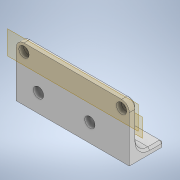
# Autodesk Inventor part: bracket_t265nd455_external
Saved by Autodesk Inventor 2022.1 (Build 261234000, 234)
## iProperties
Created: 2021-08-20
Part Number: bracket_t265nd455_external
Material: Generic
Document SubType Name: Modeling
Designer: 오유진
Density: 1 g/cm^3
Appearance: Default
Author: 오유진
Autodesk Inventor part; units mm, degrees
(part 1 of 2)
ref_plane "YZ Plane" through (0, 0, 0) normal (1, 0, 0) x (0, 1, 0)
ref_plane "XZ Plane" through (0, 0, 0) normal (0, 1, 0) x (-1, 0, 0)
ref_plane "XY Plane" through (0, 0, 0) normal (0, 0, 1) x (1, 0, 0)
ref_plane "Work Plane3" through (-46, 39.5, 21) normal (0, 0, 1) x (1, 0, 0)
sketch "Sketch5" plane through (-46, 39.5, 21) normal (0, 0, 1) x (1, 0, 0)
  line L0 (41.5, 10.3889) -> (-41.5, 10.3889) projected
  spline S0 degree 3 poles (-52.6944, 8.9971) (-52.5847, 9.0604) (-52.4738, 9.1218) (-52.3618, 9.181) (-52.263, 9.2333) (-52.1634, 9.2839) (-52.063, 9.3329) (-51.9718, 9.3773) (-51.8801, 9.4203) (-51.7876, 9.4618) (-51.6999, 9.5013) (-51.6116, 9.5395) (-51.5228, 9.5763) (-51.435, 9.6128) (-51.3468, 9.6479) (-51.258, 9.6817) (-51.1696, 9.7154) (-51.0807, 9.7479) (-50.9913, 9.779) (-50.9017, 9.8102) (-50.8117, 9.8401) (-50.7213, 9.8687) (-50.6307, 9.8973) (-50.5398, 9.9246) (-50.4485, 9.9506) (-50.3572, 9.9766) (-50.2655, 10.0013) (-50.1736, 10.0246) (-50.0816, 10.0479) (-49.9892, 10.0699) (-49.8966, 10.0905) (-49.8038, 10.1112) (-49.7107, 10.1306) (-49.6173, 10.1486) (-49.5236, 10.1666) (-49.4296, 10.1834) (-49.3352, 10.1989) (-49.2404, 10.2144) (-49.1453, 10.2287) (-49.0498, 10.2418) (-48.9539, 10.255) (-48.8576, 10.267) (-48.7611, 10.2779) (-48.6642, 10.2888) (-48.567, 10.2987) (-48.4696, 10.3076) (-48.3718, 10.3166) (-48.2737, 10.3245) (-48.1754, 10.3316) (-48.0763, 10.3388) (-47.977, 10.345) (-47.8775, 10.3505) (-47.7769, 10.3561) (-47.6762, 10.3609) (-47.5754, 10.365) (-47.4739, 10.3691) (-47.3722, 10.3726) (-47.2704, 10.3755) (-47.1677, 10.3785) (-47.065, 10.3808) (-46.9621, 10.3827) (-46.8576, 10.3847) (-46.753, 10.3862) (-46.6483, 10.3873) (-46.5422, 10.3884) (-46.436, 10.3892) (-46.3298, 10.3897) (-46.2236, 10.3902) (-46.1173, 10.3905) (-46.011, 10.3906) (-45.9052, 10.3907) (-45.7994, 10.3907) (-45.6934, 10.3906) (-45.5876, 10.3905) (-45.4817, 10.3903) (-45.3757, 10.3902) (-45.2696, 10.39) (-45.1635, 10.3899) (-45.0574, 10.3898) (-44.9513, 10.3897) (-44.8452, 10.3896) (-44.7391, 10.3896) (-44.6331, 10.3895) (-44.5271, 10.3895) (-44.4211, 10.3895) (-44.3151, 10.3894) (-44.209, 10.3894) (-44.103, 10.3894) (-43.9969, 10.3893) (-43.8907, 10.3893) (-43.7846, 10.3893) (-43.6785, 10.3892) (-43.5724, 10.3892) (-43.4663, 10.3891) (-43.3604, 10.3891) (-43.2545, 10.3891) (-43.1486, 10.389) (-43.0427, 10.389) (-42.9368, 10.389) (-42.831, 10.389) (-42.7244, 10.3889) (-42.6178, 10.3889) (-42.5112, 10.3889) (-42.4028, 10.3889) (-42.2944, 10.3889) (-42.186, 10.3889) (-42.0747, 10.3889) (-41.9634, 10.3889) (-41.8521, 10.3889) (-41.7347, 10.3889) (-41.6174, 10.3889) (-41.5, 10.3889) knots 0 0 0 0 0.033772 0.033772 0.033772 0.063568 0.063568 0.063568 0.090608 0.090608 0.090608 0.116279 0.116279 0.116279 0.141638 0.141638 0.141638 0.166894 0.166894 0.166894 0.192211 0.192211 0.192211 0.217549 0.217549 0.217549 0.242877 0.242877 0.242877 0.268207 0.268207 0.268207 0.293578 0.293578 0.293578 0.319038 0.319038 0.319038 0.344627 0.344627 0.344627 0.370358 0.370358 0.370358 0.3962 0.3962 0.3962 0.422164 0.422164 0.422164 0.448361 0.448361 0.448361 0.47483 0.47483 0.47483 0.501477 0.501477 0.501477 0.528339 0.528339 0.528339 0.555617 0.555617 0.555617 0.583244 0.583244 0.583244 0.610845 0.610845 0.610845 0.638286 0.638286 0.638286 0.665706 0.665706 0.665706 0.693157 0.693157 0.693157 0.720597 0.720597 0.720597 0.748024 0.748024 0.748024 0.775467 0.775467 0.775467 0.802931 0.802931 0.802931 0.830389 0.830389 0.830389 0.857797 0.857797 0.857797 0.885191 0.885191 0.885191 0.912774 0.912774 0.912774 0.940826 0.940826 0.940826 0.969629 0.969629 0.969629 1 1 1 1 projected
  arc A0 (-52.6944, 8.9971) -> (-52.6944, -8.9971) centre (-47.5, 0) ccw projected
  spline S1 degree 3 poles (-41.5, -10.3889) (-41.6309, -10.3889) (-41.7619, -10.3889) (-41.8928, -10.3889) (-42.0134, -10.3889) (-42.134, -10.3889) (-42.2546, -10.3889) (-42.3674, -10.3889) (-42.4802, -10.3889) (-42.593, -10.3889) (-42.7013, -10.3889) (-42.8095, -10.3889) (-42.9178, -10.389) (-43.0247, -10.389) (-43.1315, -10.389) (-43.2384, -10.3891) (-43.3448, -10.3891) (-43.4512, -10.3891) (-43.5575, -10.3892) (-43.6641, -10.3892) (-43.7706, -10.3893) (-43.8771, -10.3893) (-43.9838, -10.3893) (-44.0904, -10.3894) (-44.197, -10.3894) (-44.3036, -10.3894) (-44.4102, -10.3895) (-44.5167, -10.3895) (-44.6232, -10.3895) (-44.7297, -10.3896) (-44.8363, -10.3896) (-44.9428, -10.3897) (-45.0493, -10.3898) (-45.1557, -10.3899) (-45.2623, -10.39) (-45.3688, -10.3902) (-45.4753, -10.3903) (-45.582, -10.3905) (-45.6885, -10.3906) (-45.795, -10.3906) (-45.9015, -10.3907) (-46.008, -10.3906) (-46.1144, -10.3904) (-46.2206, -10.3902) (-46.3267, -10.3898) (-46.4327, -10.3891) (-46.5381, -10.3884) (-46.6434, -10.3875) (-46.7486, -10.3861) (-46.8525, -10.3847) (-46.9563, -10.383) (-47.06, -10.3808) (-47.1622, -10.3786) (-47.2642, -10.3759) (-47.366, -10.3726) (-47.4669, -10.3694) (-47.5677, -10.3656) (-47.6683, -10.361) (-47.7686, -10.3565) (-47.8687, -10.3513) (-47.9687, -10.3453) (-48.068, -10.3393) (-48.1671, -10.3325) (-48.266, -10.3248) (-48.3638, -10.3172) (-48.4615, -10.3087) (-48.5589, -10.2992) (-48.6558, -10.2897) (-48.7525, -10.2792) (-48.8489, -10.2677) (-48.9453, -10.2561) (-49.0414, -10.2434) (-49.1372, -10.2295) (-49.2326, -10.2156) (-49.3277, -10.2005) (-49.4226, -10.1842) (-49.5168, -10.1679) (-49.6108, -10.1503) (-49.7044, -10.1314) (-49.7979, -10.1125) (-49.891, -10.0923) (-49.9839, -10.0707) (-50.0768, -10.0491) (-50.1695, -10.0261) (-50.2617, -10.0018) (-50.354, -9.9775) (-50.4459, -9.9518) (-50.5374, -9.9249) (-50.6288, -9.8979) (-50.7199, -9.8696) (-50.8106, -9.84) (-50.9012, -9.8104) (-50.9915, -9.7794) (-51.0812, -9.7472) (-51.1709, -9.715) (-51.2601, -9.6815) (-51.3487, -9.6466) (-51.4373, -9.6119) (-51.5253, -9.5758) (-51.6129, -9.5384) (-51.701, -9.5008) (-51.7885, -9.4619) (-51.8755, -9.4218) (-51.9643, -9.3808) (-52.0524, -9.3385) (-52.1399, -9.295) (-52.2303, -9.25) (-52.32, -9.2036) (-52.4091, -9.1559) (-52.505, -9.1045) (-52.6001, -9.0515) (-52.6944, -8.9971) knots 0 0 0 0 0.033887 0.033887 0.033887 0.06509 0.06509 0.06509 0.094285 0.094285 0.094285 0.122296 0.122296 0.122296 0.149952 0.149952 0.149952 0.177479 0.177479 0.177479 0.205048 0.205048 0.205048 0.232644 0.232644 0.232644 0.260224 0.260224 0.260224 0.287779 0.287779 0.287779 0.315326 0.315326 0.315326 0.34289 0.34289 0.34289 0.370486 0.370486 0.370486 0.398102 0.398102 0.398102 0.425677 0.425677 0.425677 0.453094 0.453094 0.453094 0.480189 0.480189 0.480189 0.506871 0.506871 0.506871 0.533301 0.533301 0.533301 0.559648 0.559648 0.559648 0.585815 0.585815 0.585815 0.611699 0.611699 0.611699 0.637449 0.637449 0.637449 0.663186 0.663186 0.663186 0.688825 0.688825 0.688825 0.714314 0.714314 0.714314 0.739759 0.739759 0.739759 0.765225 0.765225 0.765225 0.790684 0.790684 0.790684 0.816132 0.816132 0.816132 0.84159 0.84159 0.84159 0.867019 0.867019 0.867019 0.892415 0.892415 0.892415 0.917983 0.917983 0.917983 0.944058 0.944058 0.944058 0.970987 0.970987 0.970987 1 1 1 1 projected
  line L1 (-41.5, -10.3889) -> (41.5, -10.3889) projected
  spline S2 degree 3 poles (52.6945, -8.9971) (52.5838, -9.0609) (52.4721, -9.1228) (52.3592, -9.1824) (52.2597, -9.2351) (52.1593, -9.286) (52.0581, -9.3352) (51.9663, -9.3799) (51.8738, -9.4232) (51.7807, -9.465) (51.6923, -9.5047) (51.6033, -9.5431) (51.5138, -9.5801) (51.4253, -9.6167) (51.3363, -9.6521) (51.2468, -9.6861) (51.1577, -9.7199) (51.0681, -9.7525) (50.978, -9.7837) (50.8876, -9.8151) (50.7968, -9.8451) (50.7056, -9.8738) (50.6142, -9.9025) (50.5224, -9.93) (50.4302, -9.956) (50.3378, -9.9822) (50.2451, -10.0069) (50.152, -10.0304) (50.0588, -10.0538) (49.9652, -10.0759) (49.8713, -10.0966) (49.7771, -10.1174) (49.6826, -10.1368) (49.5878, -10.1549) (49.4925, -10.173) (49.3969, -10.1898) (49.3009, -10.2053) (49.2043, -10.2208) (49.1074, -10.2351) (49.0102, -10.2482) (48.9122, -10.2614) (48.8139, -10.2733) (48.7154, -10.2842) (48.6164, -10.2951) (48.5171, -10.3049) (48.4176, -10.3137) (48.3176, -10.3226) (48.2174, -10.3304) (48.117, -10.3374) (48.0156, -10.3445) (47.914, -10.3506) (47.8123, -10.356) (47.7094, -10.3614) (47.6064, -10.3661) (47.5032, -10.37) (47.3996, -10.374) (47.2959, -10.3773) (47.192, -10.3801) (47.0879, -10.3828) (46.9836, -10.385) (46.8791, -10.3867) (46.7737, -10.3885) (46.6682, -10.3898) (46.5625, -10.3907) (46.4561, -10.3916) (46.3496, -10.3922) (46.243, -10.3926) (46.1368, -10.3929) (46.0306, -10.393) (45.9243, -10.393) (45.8189, -10.3929) (45.7134, -10.3927) (45.6078, -10.3925) (45.5027, -10.3923) (45.3976, -10.392) (45.2924, -10.3917) (45.1874, -10.3914) (45.0824, -10.3912) (44.9774, -10.391) (44.8727, -10.3908) (44.7681, -10.3906) (44.6634, -10.3905) (44.5592, -10.3903) (44.4551, -10.3902) (44.3509, -10.3901) (44.2471, -10.39) (44.1434, -10.3899) (44.0396, -10.3898) (43.936, -10.3897) (43.8325, -10.3897) (43.7289, -10.3896) (43.6254, -10.3895) (43.5219, -10.3894) (43.4184, -10.3893) (43.315, -10.3893) (43.2117, -10.3892) (43.1083, -10.3891) (43.005, -10.3891) (42.9017, -10.389) (42.7984, -10.389) (42.6944, -10.389) (42.5904, -10.389) (42.4865, -10.3889) (42.3807, -10.3889) (42.275, -10.3889) (42.1693, -10.3889) (42.0607, -10.3889) (41.9521, -10.3889) (41.8435, -10.3889) (41.729, -10.3889) (41.6145, -10.3889) (41.5, -10.3889) knots 0 0 0 0 0.034033 0.034033 0.034033 0.064049 0.064049 0.064049 0.091284 0.091284 0.091284 0.117145 0.117145 0.117145 0.142696 0.142696 0.142696 0.168144 0.168144 0.168144 0.193662 0.193662 0.193662 0.219234 0.219234 0.219234 0.244842 0.244842 0.244842 0.270502 0.270502 0.270502 0.296244 0.296244 0.296244 0.322113 0.322113 0.322113 0.348164 0.348164 0.348164 0.37441 0.37441 0.37441 0.40079 0.40079 0.40079 0.427301 0.427301 0.427301 0.454074 0.454074 0.454074 0.481133 0.481133 0.481133 0.508306 0.508306 0.508306 0.53556 0.53556 0.53556 0.563073 0.563073 0.563073 0.590787 0.590787 0.590787 0.618371 0.618371 0.618371 0.645713 0.645713 0.645713 0.672935 0.672935 0.672935 0.700093 0.700093 0.700093 0.727156 0.727156 0.727156 0.754106 0.754106 0.754106 0.780956 0.780956 0.780956 0.807754 0.807754 0.807754 0.834538 0.834538 0.834538 0.861282 0.861282 0.861282 0.888009 0.888009 0.888009 0.914912 0.914912 0.914912 0.94227 0.94227 0.94227 0.970367 0.970367 0.970367 1 1 1 1 projected
  arc A1 (52.6944, -8.9971) -> (52.6944, 8.9971) centre (47.5, 0) ccw projected
  spline S3 degree 3 poles (41.5, 10.3889) (41.6279, 10.3889) (41.7557, 10.3889) (41.8836, 10.3889) (42.0013, 10.3889) (42.119, 10.3889) (42.2367, 10.3889) (42.3468, 10.3889) (42.457, 10.3889) (42.5671, 10.389) (42.6727, 10.389) (42.7783, 10.389) (42.8839, 10.389) (42.9881, 10.3891) (43.0924, 10.3891) (43.1966, 10.3892) (43.3003, 10.3893) (43.404, 10.3893) (43.5077, 10.3894) (43.6116, 10.3895) (43.7155, 10.3896) (43.8193, 10.3896) (43.9236, 10.3897) (44.0278, 10.3898) (44.132, 10.3899) (44.2366, 10.39) (44.3411, 10.3901) (44.4457, 10.3902) (44.5507, 10.3903) (44.6556, 10.3905) (44.7606, 10.3906) (44.8659, 10.3908) (44.9713, 10.391) (45.0766, 10.3912) (45.1824, 10.3914) (45.2881, 10.3917) (45.3937, 10.392) (45.4998, 10.3922) (45.6059, 10.3925) (45.7118, 10.3927) (45.8182, 10.3929) (45.9245, 10.393) (46.0307, 10.3929) (46.1372, 10.3929) (46.2436, 10.3927) (46.3499, 10.3921) (46.456, 10.3916) (46.5621, 10.3908) (46.668, 10.3896) (46.7733, 10.3885) (46.8785, 10.3869) (46.9835, 10.3848) (47.0876, 10.3828) (47.1915, 10.3803) (47.2954, 10.3771) (47.3985, 10.374) (47.5015, 10.3703) (47.6044, 10.3659) (47.7068, 10.3615) (47.8092, 10.3564) (47.9114, 10.3505) (48.0127, 10.3446) (48.1139, 10.3379) (48.2149, 10.3303) (48.3148, 10.3228) (48.4145, 10.3143) (48.5139, 10.3049) (48.6127, 10.2954) (48.7114, 10.285) (48.8097, 10.2734) (48.9079, 10.2619) (49.0058, 10.2492) (49.1034, 10.2353) (49.2004, 10.2214) (49.2971, 10.2063) (49.3935, 10.1899) (49.4892, 10.1736) (49.5846, 10.156) (49.6796, 10.137) (49.7743, 10.118) (49.8687, 10.0977) (49.9628, 10.076) (50.0568, 10.0543) (50.1505, 10.0312) (50.2438, 10.0068) (50.337, 9.9824) (50.4298, 9.9566) (50.5222, 9.9295) (50.6144, 9.9025) (50.7062, 9.8741) (50.7976, 9.8444) (50.8889, 9.8146) (50.9799, 9.7836) (51.0703, 9.7512) (51.1607, 9.7188) (51.2506, 9.6851) (51.3399, 9.6501) (51.4292, 9.6152) (51.5179, 9.5789) (51.6061, 9.5414) (51.6948, 9.5036) (51.783, 9.4645) (51.8706, 9.4241) (51.96, 9.3829) (52.0487, 9.3404) (52.1368, 9.2965) (52.2277, 9.2513) (52.318, 9.2047) (52.4076, 9.1567) (52.504, 9.105) (52.5996, 9.0518) (52.6944, 8.9971) knots 0 0 0 0 0.033087 0.033087 0.033087 0.063549 0.063549 0.063549 0.092041 0.092041 0.092041 0.119366 0.119366 0.119366 0.146335 0.146335 0.146335 0.173165 0.173165 0.173165 0.200045 0.200045 0.200045 0.227014 0.227014 0.227014 0.254073 0.254073 0.254073 0.281222 0.281222 0.281222 0.308465 0.308465 0.308465 0.335809 0.335809 0.335809 0.363265 0.363265 0.363265 0.390837 0.390837 0.390837 0.418478 0.418478 0.418478 0.446085 0.446085 0.446085 0.473523 0.473523 0.473523 0.500706 0.500706 0.500706 0.527712 0.527712 0.527712 0.554622 0.554622 0.554622 0.581324 0.581324 0.581324 0.607726 0.607726 0.607726 0.63397 0.63397 0.63397 0.660167 0.660167 0.660167 0.686219 0.686219 0.686219 0.712071 0.712071 0.712071 0.737837 0.737837 0.737837 0.763587 0.763587 0.763587 0.789281 0.789281 0.789281 0.814924 0.814924 0.814924 0.840566 0.840566 0.840566 0.866183 0.866183 0.866183 0.891763 0.891763 0.891763 0.917506 0.917506 0.917506 0.943749 0.943749 0.943749 0.970834 0.970834 0.970834 1 1 1 1 projected
  circle A2 centre (47.5, 0) radius 2.408 projected
  circle A3 centre (-47.5, 0) radius 2.408 projected
  circle A4 centre (-47.5, 0) radius 7.5
  circle A5 centre (47.5, 0) radius 7.5
  line L2 (-47.5, 7.5) -> (47.5, 7.5)
  spline S4 degree 3 poles (40.7, -19.15) (40.7514, -19.15) (40.7969, -19.1502) (40.8369, -19.1505) (40.8936, -19.151) (40.9392, -19.1519) (40.9764, -19.1528) (41.008, -19.1536) (41.0335, -19.1546) (41.0542, -19.1555) (41.0749, -19.1564) (41.0908, -19.1572) (41.1031, -19.158) (41.1257, -19.1594) (41.1361, -19.1603) (41.1432, -19.1612) (41.1503, -19.1621) (41.1541, -19.1631) (41.1627, -19.1661) (41.1721, -19.1694) (41.1872, -19.1753) (41.2068, -19.1846) (41.2263, -19.1938) (41.2503, -19.2064) (41.2773, -19.2229) (41.3063, -19.2405) (41.3389, -19.2625) (41.3732, -19.2879) (41.4074, -19.3134) (41.4433, -19.3422) (41.4784, -19.373) (41.498, -19.3902) (41.5174, -19.408) (41.5363, -19.4263) (41.5553, -19.4446) (41.5738, -19.4633) (41.5917, -19.4824) (41.6097, -19.5015) (41.6271, -19.521) (41.6439, -19.5406) (41.6607, -19.5603) (41.6768, -19.5802) (41.6922, -19.6001) (41.722, -19.639) (41.7489, -19.678) (41.7703, -19.7129) (41.781, -19.7303) (41.7904, -19.7467) (41.7982, -19.7609) (41.8059, -19.775) (41.8121, -19.787) (41.8168, -19.7962) (41.8248, -19.8119) (41.8284, -19.8195) (41.831, -19.8259) (41.8335, -19.8322) (41.8351, -19.8374) (41.837, -19.8498) (41.8383, -19.8587) (41.8399, -19.8713) (41.8414, -19.8899) (41.843, -19.9086) (41.8445, -19.9334) (41.8458, -19.967) (41.8473, -20.0055) (41.8485, -20.0556) (41.8492, -20.1223) (41.8497, -20.1721) (41.85, -20.2311) (41.85, -20.3) knots 0 0 0 0 0.023446 0.023446 0.023446 0.056675 0.056675 0.056675 0.085016 0.085016 0.085016 0.113357 0.113357 0.113357 0.165377 0.165377 0.165377 0.217397 0.217397 0.217397 0.274605 0.274605 0.274605 0.331813 0.331813 0.331813 0.393015 0.393015 0.393015 0.454218 0.454218 0.454218 0.488473 0.488473 0.488473 0.522729 0.522729 0.522729 0.556985 0.556985 0.556985 0.591241 0.591241 0.591241 0.657881 0.657881 0.657881 0.6912 0.6912 0.6912 0.72452 0.72452 0.72452 0.781391 0.781391 0.781391 0.838262 0.838262 0.838262 0.878699 0.878699 0.878699 0.919137 0.919137 0.919137 0.965453 0.965453 0.965453 1 1 1 1 projected
  line L3 (40.7, -19.15) -> (-56.7, -19.15) projected
  spline S5 degree 3 poles (-57.85, -20.3) (-57.85, -20.2486) (-57.8498, -20.2031) (-57.8495, -20.1631) (-57.849, -20.1064) (-57.8481, -20.0608) (-57.8472, -20.0236) (-57.8464, -19.992) (-57.8454, -19.9665) (-57.8445, -19.9458) (-57.8436, -19.9251) (-57.8428, -19.9092) (-57.842, -19.8969) (-57.8406, -19.8743) (-57.8397, -19.8639) (-57.8388, -19.8568) (-57.8379, -19.8497) (-57.8369, -19.8459) (-57.8339, -19.8373) (-57.8306, -19.8279) (-57.8247, -19.8128) (-57.8154, -19.7932) (-57.8062, -19.7737) (-57.7936, -19.7497) (-57.7771, -19.7227) (-57.7595, -19.6937) (-57.7375, -19.6611) (-57.7121, -19.6268) (-57.6866, -19.5926) (-57.6578, -19.5567) (-57.627, -19.5216) (-57.6098, -19.502) (-57.592, -19.4826) (-57.5737, -19.4637) (-57.5554, -19.4447) (-57.5367, -19.4262) (-57.5176, -19.4083) (-57.4985, -19.3903) (-57.479, -19.3729) (-57.4594, -19.3561) (-57.4397, -19.3393) (-57.4198, -19.3232) (-57.3999, -19.3078) (-57.361, -19.278) (-57.322, -19.2511) (-57.2871, -19.2297) (-57.2697, -19.219) (-57.2533, -19.2096) (-57.2391, -19.2018) (-57.225, -19.1941) (-57.213, -19.1879) (-57.2038, -19.1832) (-57.1881, -19.1752) (-57.1805, -19.1716) (-57.1741, -19.169) (-57.1678, -19.1665) (-57.1626, -19.1649) (-57.1502, -19.163) (-57.1413, -19.1617) (-57.1287, -19.1601) (-57.1101, -19.1586) (-57.0914, -19.157) (-57.0666, -19.1555) (-57.033, -19.1542) (-56.9945, -19.1527) (-56.9444, -19.1515) (-56.8777, -19.1508) (-56.8279, -19.1503) (-56.7689, -19.15) (-56.7, -19.15) knots 0 0 0 0 0.023446 0.023446 0.023446 0.056675 0.056675 0.056675 0.085016 0.085016 0.085016 0.113357 0.113357 0.113357 0.165377 0.165377 0.165377 0.217397 0.217397 0.217397 0.274605 0.274605 0.274605 0.331813 0.331813 0.331813 0.393015 0.393015 0.393015 0.454218 0.454218 0.454218 0.488473 0.488473 0.488473 0.522729 0.522729 0.522729 0.556985 0.556985 0.556985 0.591241 0.591241 0.591241 0.657881 0.657881 0.657881 0.6912 0.6912 0.6912 0.72452 0.72452 0.72452 0.781391 0.781391 0.781391 0.838262 0.838262 0.838262 0.878699 0.878699 0.878699 0.919137 0.919137 0.919137 0.965453 0.965453 0.965453 1 1 1 1 projected
  line L4 (-57.85, -20.3) -> (-57.85, -34.2) projected
  spline S6 degree 3 poles (-56.7, -35.35) (-56.7514, -35.35) (-56.7969, -35.3498) (-56.8369, -35.3495) (-56.8936, -35.349) (-56.9392, -35.3481) (-56.9764, -35.3472) (-57.008, -35.3464) (-57.0335, -35.3454) (-57.0542, -35.3445) (-57.0749, -35.3436) (-57.0908, -35.3428) (-57.1031, -35.342) (-57.1257, -35.3406) (-57.1361, -35.3397) (-57.1432, -35.3388) (-57.1503, -35.3379) (-57.1541, -35.3369) (-57.1627, -35.3339) (-57.1721, -35.3306) (-57.1872, -35.3247) (-57.2068, -35.3154) (-57.2263, -35.3062) (-57.2503, -35.2936) (-57.2773, -35.2771) (-57.3063, -35.2595) (-57.3389, -35.2375) (-57.3732, -35.2121) (-57.4074, -35.1866) (-57.4433, -35.1578) (-57.4784, -35.127) (-57.498, -35.1098) (-57.5174, -35.092) (-57.5363, -35.0737) (-57.5553, -35.0554) (-57.5738, -35.0367) (-57.5917, -35.0176) (-57.6097, -34.9985) (-57.6271, -34.979) (-57.6439, -34.9594) (-57.6607, -34.9397) (-57.6768, -34.9198) (-57.6922, -34.8999) (-57.722, -34.861) (-57.7489, -34.822) (-57.7703, -34.7871) (-57.781, -34.7697) (-57.7904, -34.7533) (-57.7982, -34.7391) (-57.8059, -34.725) (-57.8121, -34.713) (-57.8168, -34.7038) (-57.8248, -34.6881) (-57.8284, -34.6805) (-57.831, -34.6741) (-57.8335, -34.6678) (-57.8351, -34.6626) (-57.837, -34.6502) (-57.8383, -34.6413) (-57.8399, -34.6287) (-57.8414, -34.6101) (-57.843, -34.5914) (-57.8445, -34.5666) (-57.8458, -34.533) (-57.8473, -34.4945) (-57.8485, -34.4444) (-57.8492, -34.3777) (-57.8497, -34.3279) (-57.85, -34.2689) (-57.85, -34.2) knots 0 0 0 0 0.023446 0.023446 0.023446 0.056675 0.056675 0.056675 0.085016 0.085016 0.085016 0.113357 0.113357 0.113357 0.165377 0.165377 0.165377 0.217397 0.217397 0.217397 0.274605 0.274605 0.274605 0.331813 0.331813 0.331813 0.393015 0.393015 0.393015 0.454218 0.454218 0.454218 0.488473 0.488473 0.488473 0.522729 0.522729 0.522729 0.556985 0.556985 0.556985 0.591241 0.591241 0.591241 0.657881 0.657881 0.657881 0.6912 0.6912 0.6912 0.72452 0.72452 0.72452 0.781391 0.781391 0.781391 0.838262 0.838262 0.838262 0.878699 0.878699 0.878699 0.919137 0.919137 0.919137 0.965453 0.965453 0.965453 1 1 1 1 projected
  line L5 (-56.7, -35.35) -> (40.7, -35.35) projected
  spline S7 degree 3 poles (41.85, -34.2) (41.85, -34.2514) (41.8498, -34.2969) (41.8495, -34.3369) (41.849, -34.3936) (41.8481, -34.4392) (41.8472, -34.4764) (41.8464, -34.508) (41.8454, -34.5335) (41.8445, -34.5542) (41.8436, -34.5749) (41.8428, -34.5908) (41.842, -34.6031) (41.8406, -34.6257) (41.8397, -34.6361) (41.8388, -34.6432) (41.8379, -34.6503) (41.8369, -34.6541) (41.8339, -34.6627) (41.8306, -34.6721) (41.8247, -34.6872) (41.8154, -34.7068) (41.8062, -34.7263) (41.7936, -34.7503) (41.7771, -34.7773) (41.7595, -34.8063) (41.7375, -34.8389) (41.7121, -34.8732) (41.6866, -34.9074) (41.6578, -34.9433) (41.627, -34.9784) (41.6098, -34.998) (41.592, -35.0174) (41.5737, -35.0363) (41.5554, -35.0553) (41.5367, -35.0738) (41.5176, -35.0917) (41.4985, -35.1097) (41.479, -35.1271) (41.4594, -35.1439) (41.4397, -35.1607) (41.4198, -35.1768) (41.3999, -35.1922) (41.361, -35.222) (41.322, -35.2489) (41.2871, -35.2703) (41.2697, -35.281) (41.2533, -35.2904) (41.2391, -35.2982) (41.225, -35.3059) (41.213, -35.3121) (41.2038, -35.3168) (41.1881, -35.3248) (41.1805, -35.3284) (41.1741, -35.331) (41.1678, -35.3335) (41.1626, -35.3351) (41.1502, -35.337) (41.1413, -35.3383) (41.1287, -35.3399) (41.1101, -35.3414) (41.0914, -35.343) (41.0666, -35.3445) (41.033, -35.3458) (40.9945, -35.3473) (40.9444, -35.3485) (40.8777, -35.3492) (40.8279, -35.3497) (40.7689, -35.35) (40.7, -35.35) knots 0 0 0 0 0.023446 0.023446 0.023446 0.056675 0.056675 0.056675 0.085016 0.085016 0.085016 0.113357 0.113357 0.113357 0.165377 0.165377 0.165377 0.217397 0.217397 0.217397 0.274605 0.274605 0.274605 0.331813 0.331813 0.331813 0.393015 0.393015 0.393015 0.454218 0.454218 0.454218 0.488473 0.488473 0.488473 0.522729 0.522729 0.522729 0.556985 0.556985 0.556985 0.591241 0.591241 0.591241 0.657881 0.657881 0.657881 0.6912 0.6912 0.6912 0.72452 0.72452 0.72452 0.781391 0.781391 0.781391 0.838262 0.838262 0.838262 0.878699 0.878699 0.878699 0.919137 0.919137 0.919137 0.965453 0.965453 0.965453 1 1 1 1 projected
  line L6 (41.85, -34.2) -> (41.85, -20.3) projected
  circle A6 centre (-33.35, -27.25) radius 1.25 projected
  circle A7 centre (16.65, -27.25) radius 1.25 projected
  line L7 (-55, 0) -> (-55, -45)
  line L8 (-55, -45) -> (55, -45)
  line L9 (55, -45) -> (55, 0)
  point P0 (46, -39.5)
  dimension "d2" = 15
  dimension "d3" = 15
  dimension "d4" = 45
  constraints: 8 end point, 4 point on circle, 3 perpendicular, 2 centre point, 2 coincident, 2 tangent, 1 parallel
  measures "d2" diameter of A4
  measures "d3" diameter of A5
  measures "d4" distance of L7.start L7.end
extrude "Extrusion1" add sketch "Sketch5" against normal blind 7.5 contours L9 L8 L7 L5 S7 L6 S4 L3 A0 S1 L1 S2 A1 | A1 S2 L1 S1 A0 L7 A4 L2 A5 L9 | A5 | A4 | L3 S4 L6 S7 L5 L7 | A2 | A3 | A6 | A7
ref_plane "Work Plane4" through (0, 0, 0) normal (0, 0, 1) x (1, 0, 0)
sketch "Sketch6" plane through (0, 0, 0) normal (0, 0, 1) x (1, 0, 0)
  spline S0 degree 3 poles (-5.3, 20.35) (-5.2486, 20.35) (-5.2031, 20.3498) (-5.1631, 20.3495) (-5.1064, 20.349) (-5.0608, 20.3481) (-5.0236, 20.3472) (-4.992, 20.3464) (-4.9665, 20.3454) (-4.9458, 20.3445) (-4.9251, 20.3436) (-4.9092, 20.3428) (-4.8969, 20.342) (-4.8743, 20.3406) (-4.8639, 20.3397) (-4.8568, 20.3388) (-4.8497, 20.3379) (-4.8459, 20.3369) (-4.8373, 20.3339) (-4.8279, 20.3306) (-4.8128, 20.3247) (-4.7932, 20.3154) (-4.7737, 20.3062) (-4.7497, 20.2936) (-4.7227, 20.2771) (-4.6937, 20.2595) (-4.6611, 20.2375) (-4.6268, 20.2121) (-4.5926, 20.1866) (-4.5567, 20.1578) (-4.5216, 20.127) (-4.502, 20.1098) (-4.4826, 20.092) (-4.4637, 20.0737) (-4.4447, 20.0554) (-4.4262, 20.0367) (-4.4083, 20.0176) (-4.3903, 19.9985) (-4.3729, 19.979) (-4.3561, 19.9594) (-4.3393, 19.9397) (-4.3232, 19.9198) (-4.3078, 19.8999) (-4.278, 19.861) (-4.2511, 19.822) (-4.2297, 19.7871) (-4.219, 19.7697) (-4.2096, 19.7533) (-4.2018, 19.7391) (-4.1941, 19.725) (-4.1879, 19.713) (-4.1832, 19.7038) (-4.1752, 19.6881) (-4.1716, 19.6805) (-4.169, 19.6741) (-4.1665, 19.6678) (-4.1649, 19.6626) (-4.163, 19.6502) (-4.1617, 19.6413) (-4.1601, 19.6287) (-4.1586, 19.6101) (-4.157, 19.5914) (-4.1555, 19.5666) (-4.1542, 19.533) (-4.1527, 19.4945) (-4.1515, 19.4444) (-4.1508, 19.3777) (-4.1503, 19.3279) (-4.15, 19.2689) (-4.15, 19.2) knots 0 0 0 0 0.023446 0.023446 0.023446 0.056675 0.056675 0.056675 0.085016 0.085016 0.085016 0.113357 0.113357 0.113357 0.165377 0.165377 0.165377 0.217397 0.217397 0.217397 0.274605 0.274605 0.274605 0.331813 0.331813 0.331813 0.393015 0.393015 0.393015 0.454218 0.454218 0.454218 0.488473 0.488473 0.488473 0.522729 0.522729 0.522729 0.556985 0.556985 0.556985 0.591241 0.591241 0.591241 0.657881 0.657881 0.657881 0.6912 0.6912 0.6912 0.72452 0.72452 0.72452 0.781391 0.781391 0.781391 0.838262 0.838262 0.838262 0.878699 0.878699 0.878699 0.919137 0.919137 0.919137 0.965453 0.965453 0.965453 1 1 1 1 projected
  line L0 (-5.3, 20.35) -> (-102.7, 20.35) projected
  spline S1 degree 3 poles (-103.85, 19.2) (-103.85, 19.2514) (-103.8498, 19.2969) (-103.8495, 19.3369) (-103.849, 19.3936) (-103.8481, 19.4392) (-103.8472, 19.4764) (-103.8464, 19.508) (-103.8454, 19.5335) (-103.8445, 19.5542) (-103.8436, 19.5749) (-103.8428, 19.5908) (-103.842, 19.6031) (-103.8406, 19.6257) (-103.8397, 19.6361) (-103.8388, 19.6432) (-103.8379, 19.6503) (-103.8369, 19.6541) (-103.8339, 19.6627) (-103.8306, 19.6721) (-103.8247, 19.6872) (-103.8154, 19.7068) (-103.8062, 19.7263) (-103.7936, 19.7503) (-103.7771, 19.7773) (-103.7595, 19.8063) (-103.7375, 19.8389) (-103.7121, 19.8732) (-103.6866, 19.9074) (-103.6578, 19.9433) (-103.627, 19.9784) (-103.6098, 19.998) (-103.592, 20.0174) (-103.5737, 20.0363) (-103.5554, 20.0553) (-103.5367, 20.0738) (-103.5176, 20.0917) (-103.4985, 20.1097) (-103.479, 20.1271) (-103.4594, 20.1439) (-103.4397, 20.1607) (-103.4198, 20.1768) (-103.3999, 20.1922) (-103.361, 20.222) (-103.322, 20.2489) (-103.2871, 20.2703) (-103.2697, 20.281) (-103.2533, 20.2904) (-103.2391, 20.2982) (-103.225, 20.3059) (-103.213, 20.3121) (-103.2038, 20.3168) (-103.1881, 20.3248) (-103.1805, 20.3284) (-103.1741, 20.331) (-103.1678, 20.3335) (-103.1626, 20.3351) (-103.1502, 20.337) (-103.1413, 20.3383) (-103.1287, 20.3399) (-103.1101, 20.3414) (-103.0914, 20.343) (-103.0666, 20.3445) (-103.033, 20.3458) (-102.9945, 20.3473) (-102.9444, 20.3485) (-102.8777, 20.3492) (-102.8279, 20.3497) (-102.7689, 20.35) (-102.7, 20.35) knots 0 0 0 0 0.023446 0.023446 0.023446 0.056675 0.056675 0.056675 0.085016 0.085016 0.085016 0.113357 0.113357 0.113357 0.165377 0.165377 0.165377 0.217397 0.217397 0.217397 0.274605 0.274605 0.274605 0.331813 0.331813 0.331813 0.393015 0.393015 0.393015 0.454218 0.454218 0.454218 0.488473 0.488473 0.488473 0.522729 0.522729 0.522729 0.556985 0.556985 0.556985 0.591241 0.591241 0.591241 0.657881 0.657881 0.657881 0.6912 0.6912 0.6912 0.72452 0.72452 0.72452 0.781391 0.781391 0.781391 0.838262 0.838262 0.838262 0.878699 0.878699 0.878699 0.919137 0.919137 0.919137 0.965453 0.965453 0.965453 1 1 1 1 projected
  line L1 (-103.85, 19.2) -> (-103.85, 5.3) projected
  spline S2 degree 3 poles (-102.7, 4.15) (-102.7514, 4.15) (-102.7969, 4.1502) (-102.8369, 4.1505) (-102.8936, 4.151) (-102.9392, 4.1519) (-102.9764, 4.1528) (-103.008, 4.1536) (-103.0335, 4.1546) (-103.0542, 4.1555) (-103.0749, 4.1564) (-103.0908, 4.1572) (-103.1031, 4.158) (-103.1257, 4.1594) (-103.1361, 4.1603) (-103.1432, 4.1612) (-103.1503, 4.1621) (-103.1541, 4.1631) (-103.1627, 4.1661) (-103.1721, 4.1694) (-103.1872, 4.1753) (-103.2068, 4.1846) (-103.2263, 4.1938) (-103.2503, 4.2064) (-103.2773, 4.2229) (-103.3063, 4.2405) (-103.3389, 4.2625) (-103.3732, 4.2879) (-103.4074, 4.3134) (-103.4433, 4.3422) (-103.4784, 4.373) (-103.498, 4.3902) (-103.5174, 4.408) (-103.5363, 4.4263) (-103.5553, 4.4446) (-103.5738, 4.4633) (-103.5917, 4.4824) (-103.6097, 4.5015) (-103.6271, 4.521) (-103.6439, 4.5406) (-103.6607, 4.5603) (-103.6768, 4.5802) (-103.6922, 4.6001) (-103.722, 4.639) (-103.7489, 4.678) (-103.7703, 4.7129) (-103.781, 4.7303) (-103.7904, 4.7467) (-103.7982, 4.7609) (-103.8059, 4.775) (-103.8121, 4.787) (-103.8168, 4.7962) (-103.8248, 4.8119) (-103.8284, 4.8195) (-103.831, 4.8259) (-103.8335, 4.8322) (-103.8351, 4.8374) (-103.837, 4.8498) (-103.8383, 4.8587) (-103.8399, 4.8713) (-103.8414, 4.8899) (-103.843, 4.9086) (-103.8445, 4.9334) (-103.8458, 4.967) (-103.8473, 5.0055) (-103.8485, 5.0556) (-103.8492, 5.1223) (-103.8497, 5.1721) (-103.85, 5.2311) (-103.85, 5.3) knots 0 0 0 0 0.023446 0.023446 0.023446 0.056675 0.056675 0.056675 0.085016 0.085016 0.085016 0.113357 0.113357 0.113357 0.165377 0.165377 0.165377 0.217397 0.217397 0.217397 0.274605 0.274605 0.274605 0.331813 0.331813 0.331813 0.393015 0.393015 0.393015 0.454218 0.454218 0.454218 0.488473 0.488473 0.488473 0.522729 0.522729 0.522729 0.556985 0.556985 0.556985 0.591241 0.591241 0.591241 0.657881 0.657881 0.657881 0.6912 0.6912 0.6912 0.72452 0.72452 0.72452 0.781391 0.781391 0.781391 0.838262 0.838262 0.838262 0.878699 0.878699 0.878699 0.919137 0.919137 0.919137 0.965453 0.965453 0.965453 1 1 1 1 projected
  line L2 (-102.7, 4.15) -> (-5.3, 4.15) projected
  spline S3 degree 3 poles (-4.15, 5.3) (-4.15, 5.2486) (-4.1502, 5.2031) (-4.1505, 5.1631) (-4.151, 5.1064) (-4.1519, 5.0608) (-4.1528, 5.0236) (-4.1536, 4.992) (-4.1546, 4.9665) (-4.1555, 4.9458) (-4.1564, 4.9251) (-4.1572, 4.9092) (-4.158, 4.8969) (-4.1594, 4.8743) (-4.1603, 4.8639) (-4.1612, 4.8568) (-4.1621, 4.8497) (-4.1631, 4.8459) (-4.1661, 4.8373) (-4.1694, 4.8279) (-4.1753, 4.8128) (-4.1846, 4.7932) (-4.1938, 4.7737) (-4.2064, 4.7497) (-4.2229, 4.7227) (-4.2405, 4.6937) (-4.2625, 4.6611) (-4.2879, 4.6268) (-4.3134, 4.5926) (-4.3422, 4.5567) (-4.373, 4.5216) (-4.3902, 4.502) (-4.408, 4.4826) (-4.4263, 4.4637) (-4.4446, 4.4447) (-4.4633, 4.4262) (-4.4824, 4.4083) (-4.5015, 4.3903) (-4.521, 4.3729) (-4.5406, 4.3561) (-4.5603, 4.3393) (-4.5802, 4.3232) (-4.6001, 4.3078) (-4.639, 4.278) (-4.678, 4.2511) (-4.7129, 4.2297) (-4.7303, 4.219) (-4.7467, 4.2096) (-4.7609, 4.2018) (-4.775, 4.1941) (-4.787, 4.1879) (-4.7962, 4.1832) (-4.8119, 4.1752) (-4.8195, 4.1716) (-4.8259, 4.169) (-4.8322, 4.1665) (-4.8374, 4.1649) (-4.8498, 4.163) (-4.8587, 4.1617) (-4.8713, 4.1601) (-4.8899, 4.1586) (-4.9086, 4.157) (-4.9334, 4.1555) (-4.967, 4.1542) (-5.0055, 4.1527) (-5.0556, 4.1515) (-5.1223, 4.1508) (-5.1721, 4.1503) (-5.2311, 4.15) (-5.3, 4.15) knots 0 0 0 0 0.023446 0.023446 0.023446 0.056675 0.056675 0.056675 0.085016 0.085016 0.085016 0.113357 0.113357 0.113357 0.165377 0.165377 0.165377 0.217397 0.217397 0.217397 0.274605 0.274605 0.274605 0.331813 0.331813 0.331813 0.393015 0.393015 0.393015 0.454218 0.454218 0.454218 0.488473 0.488473 0.488473 0.522729 0.522729 0.522729 0.556985 0.556985 0.556985 0.591241 0.591241 0.591241 0.657881 0.657881 0.657881 0.6912 0.6912 0.6912 0.72452 0.72452 0.72452 0.781391 0.781391 0.781391 0.838262 0.838262 0.838262 0.878699 0.878699 0.878699 0.919137 0.919137 0.919137 0.965453 0.965453 0.965453 1 1 1 1 projected
  line L3 (-4.15, 5.3) -> (-4.15, 19.2) projected
  circle A0 centre (-79.35, 12.25) radius 1.25 projected
  circle A1 centre (-29.35, 12.25) radius 1.25 projected
  line L4 (9, -5.5) -> (-101, -5.5) projected
  line L5 (-101, -5.5) -> (-101, 39.5) projected
  arc A2 (-93.5, 47) -> (-101, 39.5) centre (-93.5, 39.5) ccw projected
  line L6 (-93.5, 47) -> (1.5, 47) projected
  arc A3 (9, 39.5) -> (1.5, 47) centre (1.5, 39.5) ccw projected
  line L7 (9, 39.5) -> (9, -5.5) projected
  circle A4 centre (-79.35, 12.25) radius 5
  circle A5 centre (-29.35, 12.25) radius 5
  line L8 (-84.35, 17.25) -> (-74.35, 17.25)
  line L9 (-74.35, 17.25) -> (-74.35, -0.25)
  line L10 (-74.35, -0.25) -> (-84.35, -0.25)
  line L11 (-84.35, -0.25) -> (-84.35, 17.25)
  line L12 (-34.35, 17.25) -> (-24.35, 17.25)
  line L13 (-24.35, 17.25) -> (-24.35, -0.25)
  line L14 (-24.35, -0.25) -> (-34.35, -0.25)
  line L15 (-34.35, -0.25) -> (-34.35, 17.25)
  point P0 (0, 0)
  dimension "d12" = 10
  dimension "d13" = 10
  dimension "d14" = 17.5
  constraints: 16 end point, 4 parallel, 2 centre point, 2 coincident, 2 horizontal, 2 perpendicular, 2 point on line
  measures "d12" diameter of A4
  measures "d13" diameter of A5
  measures "d14" distance of L8.end L9.end
extrude "Extrusion2" add sketch "Sketch6" along normal blind 13.5 contours L11 A4 L9 L2 | L2 L9 L10 L11 | L13 L14 L15 L2 | L2 L15 A5 L13 | L11 L8 A4 | A4 | A5 | A5 L12 L13 | A4 L8 L9 | L15 L12 A5 | A0 | A1
sketch "Sketch9" plane through (-46, 39.5, 13.5) normal (0, 0, -1) x (-1, 0, 0)
  line L0 (-11.65, -39.75) -> (-21.65, -39.75) projected
  line L1 (-21.65, -39.75) -> (-21.65, -22.25) projected
  line L2 (-21.65, -22.25) -> (-11.65, -22.25) projected
  line L3 (-11.65, -22.25) -> (-11.65, -39.75) projected
  line L4 (38.35, -39.75) -> (28.35, -39.75) projected
  line L5 (28.35, -39.75) -> (28.35, -22.25) projected
  line L6 (28.35, -22.25) -> (38.35, -22.25) projected
  line L7 (38.35, -22.25) -> (38.35, -39.75) projected
  line L8 (-55, -45) -> (55, -45) projected
  line L9 (55, -45) -> (55, 0) projected
  arc A0 (55, 0) -> (47.5, 7.5) centre (47.5, 0) ccw projected
  line L10 (47.5, 7.5) -> (-47.5, 7.5) projected
  arc A1 (-47.5, 7.5) -> (-55, 0) centre (-47.5, 0) ccw projected
  line L11 (-55, 0) -> (-55, -45) projected
  line L12 (-40.7, -39.5) -> (56.7, -39.5) projected
  spline S0 degree 3 poles (-40.7, -39.5) (-41.0039, -39.5) (-41.6148, -39.4956) (-42.5911, -39.276) (-43.5888, -38.7751) (-44.5183, -38.0183) (-45.2751, -37.0888) (-45.776, -36.0911) (-45.9956, -35.1148) (-46, -34.5039) (-46, -34.2) knots 0 0 0 0 0.125 0.25 0.375 0.5 0.625 0.75 0.875 1 1 1 1 projected
  line L13 (-46, -20.3) -> (-46, -34.2) projected
  spline S1 degree 3 poles (-46, -20.3) (-46, -19.9961) (-45.9956, -19.3852) (-45.776, -18.4089) (-45.2751, -17.4112) (-44.5183, -16.4817) (-43.5888, -15.7249) (-42.5911, -15.224) (-41.6148, -15.0044) (-41.0039, -15) (-40.7, -15) knots 0 0 0 0 0.125 0.25 0.375 0.5 0.625 0.75 0.875 1 1 1 1 projected
  spline S2 degree 3 poles (62, -34.2) (62, -34.5039) (61.9956, -35.1148) (61.776, -36.0911) (61.2751, -37.0888) (60.5183, -38.0183) (59.5888, -38.7751) (58.5911, -39.276) (57.6148, -39.4956) (57.0039, -39.5) (56.7, -39.5) knots 0 0 0 0 0.125 0.25 0.375 0.5 0.625 0.75 0.875 1 1 1 1 projected
  line L14 (62, -34.2) -> (62, -20.3) projected
  spline S3 degree 3 poles (56.7, -15) (57.0039, -15) (57.6148, -15.0044) (58.5911, -15.224) (59.5888, -15.7249) (60.5183, -16.4817) (61.2751, -17.4112) (61.776, -18.4089) (61.9956, -19.3852) (62, -19.9961) (62, -20.3) knots 0 0 0 0 0.125 0.25 0.375 0.5 0.625 0.75 0.875 1 1 1 1 projected
  line L15 (56.7, -15) -> (-40.7, -15) projected
  line L16 (-55, 0) -> (-55, -45) projected
  line L17 (-55, -39.75) -> (55, -39.75)
  line L18 (55, -45) -> (55, 0) projected
  line L19 (-55, -45) -> (55, -45) projected
  line L20 (-55, -39.75) -> (-55, -45)
  line L21 (-55, -45) -> (55, -45)
  line L22 (55, -45) -> (55, -39.75)
  point P0 (-46, -39.5)
  point P1 (55, -39.75)
  point P2 (-11.65, -39.75)
  point P3 (-21.65, -39.75)
  constraints: 8 end point, 2 collinear, 2 point on line, 1 horizontal, 1 perpendicular
extrude "Extrusion4" add sketch "Sketch9" along normal blind 26 contours L17 L4 L9 L8 L11 L0
fillet "Fillet1" radius 12.5 3 edges at (-7.675, -0.25, 13.5) (-54.35, -0.25, 13.5) (-92.675, -0.25, 13.5)
fillet "Fillet2" radius 7.5 2 edges at (-29.35, 17.25, 13.5) (-79.35, 17.25, 13.5)
chamfer "Chamfer1" distance 2 angle 45 14 edges at (9, -2.875, -12.5) (-101, -2.875, -12.5) (-79.35, 17.25, 0) (-29.35, 17.25, 0) (6.8033, 44.8033, 13.5) (9, 25.875, 13.5) (9, 3.4112, 9.8388) (9, -0.25, -5.75) (-46, 47, 13.5) (-98.8033, 44.8033, 13.5) (-101, 25.875, 13.5) (-101, 3.4112, 9.8388) (-101, -0.25, -5.75) (-46, -0.25, -12.5)